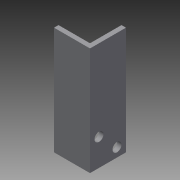
# Autodesk Inventor part: 1x1 angle mechanical stop
Saved by Autodesk Inventor 2015 SP1 (Build 190203100, 203)
## iProperties
Created: 2015-01-27
Part Number: 1x1 angle mechanical stop
Material: Generic
Document SubType Name: Modeling
Designer: Admin
Density: 1 g/cm^3
Appearance: Default
Author: Admin
Autodesk Inventor part; units mm, degrees
ref_plane "YZ Plane" through (0, 0, 0) normal (1, 0, 0) x (0, 1, 0)
ref_plane "XZ Plane" through (0, 0, 0) normal (0, 1, 0) x (-1, 0, 0)
ref_plane "XY Plane" through (0, 0, 0) normal (0, 0, 1) x (1, 0, 0)
sketch "Sketch1" plane through (0, 0, 0) normal (0, 1, 0) x (-1, 0, 0)
  line L0 (0, 0) -> (25.4, 0)
  line L1 (25.4, 0) -> (25.4, -3.175)
  line L2 (25.4, -3.175) -> (0, -3.175)
  line L3 (0, -3.175) -> (0, 0)
  line L4 (0, 0) -> (3.175, 0)
  line L5 (3.175, 0) -> (3.175, -25.4)
  line L6 (3.175, -25.4) -> (0, -25.4)
  line L7 (0, -25.4) -> (0, 0)
  dimension "d0" = 25.4
  dimension "d1" = 3.175
  dimension "d2" = 3.175
  dimension "d3" = 25.4
  constraints: 16 end point, 4 parallel, 2 horizontal, 2 perpendicular
  measures "d0" distance of L1.end L2.end
  measures "d1" distance of L0.end L1.end
  measures "d2" distance of L5.end L6.end
  measures "d3" distance of L4.end L5.end
extrude "Extrusion1" add sketch "Sketch1" along normal blind 76.2
sketch "Sketch2" plane through (0, 0, 0) normal (1, 0, 0) x (0, 0, -1)
  line L0 (0, 0) -> (25.4, 0) projected
  line L1 (25.4, 0) -> (25.4, 76.2) projected
  point P0 (19.05, 6.35)
  point P1 (6.35, 19.05)
  dimension "d6" = 6.35
  dimension "d7" = 6.35
  dimension "d8" = 19.05
  dimension "d9" = 19.05
  measures "d6" distance from line of L0 point (19.05, 6.35)
  measures "d7" distance from line of L1 point (19.05, 6.35)
  measures "d8" distance from line of L1 point (6.35, 19.05)
  measures "d9" distance from line of L0 point (6.35, 19.05)
hole "Hole1" at (0, 6.35, -19.05) at (0, 19.05, -6.35) direction (-1, 0, 0) diameter 6.35 end through all
body "Solid1"
